Autodesk Fusion 360 part; units mm, degrees
(part 4 of 6)
  spline S137 degree 5 poles (-9.0895, 3.5778) (-9.0878, 3.5785) (-9.078, 3.5823) (-9.0601, 3.5894) (-9.0342, 3.5998) (-9.0002, 3.6135) (-8.9599, 3.6301) (-8.9196, 3.6469) (-8.8794, 3.6639) (-8.8392, 3.6811) (-8.799, 3.6985) (-8.759, 3.7161) (-8.7189, 3.734) (-8.6789, 3.752) (-8.639, 3.7703) (-8.5991, 3.7887) (-8.5592, 3.8074) (-8.5194, 3.8262) (-8.4796, 3.8453) (-8.4399, 3.8645) (-8.4002, 3.8839) (-8.3606, 3.9035) (-8.321, 3.9233) (-8.2815, 3.9432) (-8.242, 3.9634) (-8.2025, 3.9837) (-8.1631, 4.0042) (-8.1238, 4.0248) (-8.0844, 4.0457) (-8.0452, 4.0667) (-8.006, 4.0879) (-7.9668, 4.1093) (-7.9277, 4.1308) (-7.8886, 4.1525) (-7.8495, 4.1743) (-7.8105, 4.1963) (-7.7716, 4.2185) (-7.7327, 4.2409) (-7.6938, 4.2634) (-7.655, 4.286) (-7.6163, 4.3089) (-7.5776, 4.3318) (-7.5389, 4.355) (-7.5003, 4.3783) (-7.4617, 4.4017) (-7.4232, 4.4253) (-7.3847, 4.449) (-7.3539, 4.4682) (-7.3309, 4.4826) (-7.3155, 4.4922) (-7.3078, 4.497) knots 0.354152 0.354152 0.354152 0.354152 0.354152 0.354152 0.357143 0.371429 0.385714 0.4 0.414286 0.428571 0.442857 0.457143 0.471429 0.485714 0.5 0.514286 0.528571 0.542857 0.557143 0.571429 0.585714 0.6 0.614286 0.628571 0.642857 0.657143 0.671429 0.685714 0.7 0.714286 0.728571 0.742857 0.757143 0.771429 0.785714 0.8 0.814286 0.828571 0.842857 0.857143 0.871429 0.885714 0.9 0.914286 0.928571 0.942857 0.957143 0.971429 0.985714 1 1 1 1 1 1
  arc A69 (-7.3078, 4.497) -> (-7.4124, 5.2009) centre (-40, 0) ccw
  spline S138 degree 5 poles (-7.4124, 5.2009) (-7.4212, 5.2033) (-7.4386, 5.208) (-7.4649, 5.2151) (-7.4999, 5.2245) (-7.5436, 5.236) (-7.5873, 5.2474) (-7.631, 5.2586) (-7.6748, 5.2696) (-7.7185, 5.2805) (-7.7622, 5.2913) (-7.8059, 5.3018) (-7.8497, 5.3122) (-7.8934, 5.3225) (-7.9371, 5.3325) (-7.9808, 5.3424) (-8.0245, 5.3522) (-8.0682, 5.3617) (-8.1119, 5.3711) (-8.1556, 5.3803) (-8.1993, 5.3894) (-8.243, 5.3983) (-8.2867, 5.4069) (-8.3303, 5.4155) (-8.374, 5.4238) (-8.4177, 5.432) (-8.4613, 5.4399) (-8.505, 5.4477) (-8.5486, 5.4553) (-8.5922, 5.4627) (-8.6358, 5.47) (-8.6794, 5.477) (-8.723, 5.4838) (-8.7666, 5.4905) (-8.8102, 5.4969) (-8.8538, 5.5032) (-8.8973, 5.5093) (-8.9408, 5.5151) (-8.9844, 5.5207) (-9.0279, 5.5262) (-9.0713, 5.5314) (-9.1148, 5.5364) (-9.1583, 5.5412) (-9.2017, 5.5458) (-9.2451, 5.5501) (-9.2885, 5.5543) (-9.325, 5.5575) (-9.3529, 5.5599) (-9.372, 5.5615) (-9.3825, 5.5623) (-9.3843, 5.5625) knots -1 -1 -1 -1 -1 -1 -0.985714 -0.971429 -0.957143 -0.942857 -0.928571 -0.914286 -0.9 -0.885714 -0.871429 -0.857143 -0.842857 -0.828571 -0.814286 -0.8 -0.785714 -0.771429 -0.757143 -0.742857 -0.728571 -0.714286 -0.7 -0.685714 -0.671429 -0.657143 -0.642857 -0.628571 -0.614286 -0.6 -0.585714 -0.571429 -0.557143 -0.542857 -0.528571 -0.514286 -0.5 -0.485714 -0.471429 -0.457143 -0.442857 -0.428571 -0.414286 -0.4 -0.385714 -0.371429 -0.357143 -0.354152 -0.354152 -0.354152 -0.354152 -0.354152 -0.354152
  spline S139 degree 3 poles (-9.8347, 5.9639) (-9.8221, 5.9) (-9.7971, 5.8392) (-9.7252, 5.7306) (-9.679, 5.6839) (-9.5895, 5.6231) (-9.5509, 5.6036) (-9.4696, 5.5749) (-9.4273, 5.5659) (-9.3843, 5.5625) knots 0 0 0 0 0.019532 0.019532 0.039064 0.039064 0.051994 0.051994 0.064924 0.064924 0.064924 0.064924
  arc A70 (-9.8347, 5.9639) -> (-9.8512, 6.047) centre (-40, 0) ccw
  spline S140 degree 3 poles (-9.589, 6.5903) (-9.6469, 6.5606) (-9.6985, 6.5199) (-9.7832, 6.421) (-9.8155, 6.3637) (-9.8494, 6.261) (-9.8575, 6.2185) (-9.8627, 6.1324) (-9.8597, 6.0892) (-9.8512, 6.047) knots 0 0 0 0 0.019532 0.019532 0.039064 0.039064 0.051994 0.051994 0.064924 0.064924 0.064924 0.064924
  spline S141 degree 5 poles (-9.589, 6.5903) (-9.5874, 6.5912) (-9.578, 6.5959) (-9.5609, 6.6047) (-9.5361, 6.6176) (-9.5036, 6.6346) (-9.4651, 6.6551) (-9.4267, 6.6757) (-9.3883, 6.6966) (-9.35, 6.7176) (-9.3118, 6.7389) (-9.2736, 6.7604) (-9.2355, 6.7821) (-9.1975, 6.804) (-9.1595, 6.8261) (-9.1216, 6.8483) (-9.0838, 6.8708) (-9.046, 6.8934) (-9.0083, 6.9163) (-8.9707, 6.9393) (-8.9331, 6.9625) (-8.8955, 6.9859) (-8.8581, 7.0095) (-8.8207, 7.0332) (-8.7834, 7.0571) (-8.7461, 7.0812) (-8.7089, 7.1055) (-8.6718, 7.1299) (-8.6347, 7.1545) (-8.5977, 7.1792) (-8.5607, 7.2042) (-8.5238, 7.2293) (-8.487, 7.2545) (-8.4502, 7.2799) (-8.4135, 7.3055) (-8.3769, 7.3313) (-8.3403, 7.3571) (-8.3037, 7.3832) (-8.2673, 7.4094) (-8.2309, 7.4358) (-8.1945, 7.4623) (-8.1583, 7.4889) (-8.1221, 7.5157) (-8.0859, 7.5427) (-8.0498, 7.5698) (-8.0138, 7.5971) (-7.9778, 7.6245) (-7.9491, 7.6465) (-7.9276, 7.6631) (-7.9132, 7.6742) (-7.9061, 7.6798) knots 0.354152 0.354152 0.354152 0.354152 0.354152 0.354152 0.357143 0.371429 0.385714 0.4 0.414286 0.428571 0.442857 0.457143 0.471429 0.485714 0.5 0.514286 0.528571 0.542857 0.557143 0.571429 0.585714 0.6 0.614286 0.628571 0.642857 0.657143 0.671429 0.685714 0.7 0.714286 0.728571 0.742857 0.757143 0.771429 0.785714 0.8 0.814286 0.828571 0.842857 0.857143 0.871429 0.885714 0.9 0.914286 0.928571 0.942857 0.957143 0.971429 0.985714 1 1 1 1 1 1
  arc A71 (-7.9061, 7.6798) -> (-8.0791, 8.37) centre (-40, 0) ccw
  spline S142 degree 5 poles (-8.0791, 8.37) (-8.088, 8.3715) (-8.1059, 8.3745) (-8.1327, 8.379) (-8.1684, 8.3849) (-8.2131, 8.3921) (-8.2577, 8.3991) (-8.3023, 8.406) (-8.3469, 8.4127) (-8.3915, 8.4192) (-8.4361, 8.4256) (-8.4806, 8.4319) (-8.5252, 8.4379) (-8.5697, 8.4438) (-8.6142, 8.4496) (-8.6586, 8.4551) (-8.7031, 8.4605) (-8.7475, 8.4658) (-8.7919, 8.4708) (-8.8363, 8.4757) (-8.8807, 8.4804) (-8.925, 8.485) (-8.9694, 8.4894) (-9.0137, 8.4936) (-9.0579, 8.4976) (-9.1022, 8.5014) (-9.1464, 8.5051) (-9.1906, 8.5085) (-9.2348, 8.5118) (-9.2789, 8.5149) (-9.323, 8.5178) (-9.3671, 8.5206) (-9.4112, 8.5231) (-9.4552, 8.5255) (-9.4992, 8.5276) (-9.5431, 8.5296) (-9.5871, 8.5313) (-9.631, 8.5329) (-9.6748, 8.5342) (-9.7187, 8.5354) (-9.7624, 8.5363) (-9.8062, 8.537) (-9.8499, 8.5375) (-9.8936, 8.5378) (-9.9372, 8.5379) (-9.9808, 8.5378) (-10.0175, 8.5375) (-10.0454, 8.5371) (-10.0646, 8.5368) (-10.0751, 8.5366) (-10.0769, 8.5366) knots -1 -1 -1 -1 -1 -1 -0.985714 -0.971429 -0.957143 -0.942857 -0.928571 -0.914286 -0.9 -0.885714 -0.871429 -0.857143 -0.842857 -0.828571 -0.814286 -0.8 -0.785714 -0.771429 -0.757143 -0.742857 -0.728571 -0.714286 -0.7 -0.685714 -0.671429 -0.657143 -0.642857 -0.628571 -0.614286 -0.6 -0.585714 -0.571429 -0.557143 -0.542857 -0.528571 -0.514286 -0.5 -0.485714 -0.471429 -0.457143 -0.442857 -0.428571 -0.414286 -0.4 -0.385714 -0.371429 -0.357143 -0.354152 -0.354152 -0.354152 -0.354152 -0.354152 -0.354152
  spline S143 degree 3 poles (-10.5645, 8.8919) (-10.5457, 8.8296) (-10.5149, 8.7715) (-10.4327, 8.6705) (-10.3822, 8.6285) (-10.2871, 8.5767) (-10.2468, 8.5611) (-10.163, 8.5406) (-10.12, 8.5358) (-10.0769, 8.5366) knots 0 0 0 0 0.019532 0.019532 0.039064 0.039064 0.051994 0.051994 0.064924 0.064924 0.064924 0.064924
  arc A72 (-10.5645, 8.8919) -> (-10.5891, 8.973) centre (-40, 0) ccw
  spline S144 degree 3 poles (-10.3814, 9.5394) (-10.4361, 9.5042) (-10.4835, 9.4586) (-10.5581, 9.3518) (-10.5846, 9.2917) (-10.6082, 9.1861) (-10.6122, 9.143) (-10.6089, 9.0569) (-10.6017, 9.0142) (-10.5891, 8.973) knots 0 0 0 0 0.019532 0.019532 0.039064 0.039064 0.051994 0.051994 0.064924 0.064924 0.064924 0.064924
  spline S145 degree 5 poles (-10.3814, 9.5394) (-10.3799, 9.5404) (-10.371, 9.5461) (-10.3549, 9.5565) (-10.3315, 9.5717) (-10.3008, 9.5918) (-10.2645, 9.6159) (-10.2283, 9.6403) (-10.1921, 9.6648) (-10.1561, 9.6895) (-10.1201, 9.7144) (-10.0842, 9.7396) (-10.0484, 9.7649) (-10.0127, 9.7904) (-9.9771, 9.8161) (-9.9416, 9.842) (-9.9061, 9.868) (-9.8707, 9.8943) (-9.8354, 9.9207) (-9.8002, 9.9473) (-9.7651, 9.9741) (-9.7301, 10.001) (-9.6951, 10.0281) (-9.6602, 10.0554) (-9.6254, 10.0829) (-9.5907, 10.1105) (-9.556, 10.1383) (-9.5215, 10.1663) (-9.487, 10.1944) (-9.4526, 10.2226) (-9.4182, 10.2511) (-9.384, 10.2797) (-9.3498, 10.3084) (-9.3157, 10.3373) (-9.2817, 10.3664) (-9.2477, 10.3956) (-9.2138, 10.4249) (-9.1801, 10.4544) (-9.1463, 10.4841) (-9.1127, 10.5139) (-9.0791, 10.5438) (-9.0456, 10.5739) (-9.0122, 10.6041) (-8.9789, 10.6345) (-8.9456, 10.665) (-8.9124, 10.6957) (-8.8793, 10.7265) (-8.8529, 10.7512) (-8.8331, 10.7699) (-8.8199, 10.7823) (-8.8133, 10.7885) knots 0.354152 0.354152 0.354152 0.354152 0.354152 0.354152 0.357143 0.371429 0.385714 0.4 0.414286 0.428571 0.442857 0.457143 0.471429 0.485714 0.5 0.514286 0.528571 0.542857 0.557143 0.571429 0.585714 0.6 0.614286 0.628571 0.642857 0.657143 0.671429 0.685714 0.7 0.714286 0.728571 0.742857 0.757143 0.771429 0.785714 0.8 0.814286 0.828571 0.842857 0.857143 0.871429 0.885714 0.9 0.914286 0.928571 0.942857 0.957143 0.971429 0.985714 1 1 1 1 1 1
  arc A73 (-8.8133, 10.7885) -> (-9.0532, 11.4585) centre (-40, 0) ccw
  spline S146 degree 5 poles (-9.0532, 11.4585) (-9.0623, 11.4591) (-9.0803, 11.4603) (-9.1074, 11.4622) (-9.1436, 11.4645) (-9.1887, 11.4673) (-9.2338, 11.4699) (-9.2789, 11.4724) (-9.3239, 11.4747) (-9.3689, 11.4769) (-9.4139, 11.4789) (-9.4589, 11.4807) (-9.5038, 11.4824) (-9.5487, 11.4839) (-9.5935, 11.4852) (-9.6383, 11.4864) (-9.6831, 11.4874) (-9.7278, 11.4883) (-9.7725, 11.489) (-9.8171, 11.4895) (-9.8618, 11.4898) (-9.9063, 11.49) (-9.9509, 11.49) (-9.9954, 11.4898) (-10.0398, 11.4895) (-10.0842, 11.489) (-10.1286, 11.4883) (-10.1729, 11.4874) (-10.2172, 11.4864) (-10.2614, 11.4851) (-10.3056, 11.4837) (-10.3498, 11.4821) (-10.3939, 11.4803) (-10.4379, 11.4783) (-10.4819, 11.4762) (-10.5258, 11.4738) (-10.5697, 11.4712) (-10.6136, 11.4685) (-10.6574, 11.4655) (-10.7011, 11.4624) (-10.7447, 11.459) (-10.7884, 11.4554) (-10.8319, 11.4517) (-10.8754, 11.4477) (-10.9188, 11.4435) (-10.9622, 11.4391) (-10.9987, 11.4351) (-11.0264, 11.432) (-11.0455, 11.4299) (-11.056, 11.4286) (-11.0578, 11.4284) knots -1 -1 -1 -1 -1 -1 -0.985714 -0.971429 -0.957143 -0.942857 -0.928571 -0.914286 -0.9 -0.885714 -0.871429 -0.857143 -0.842857 -0.828571 -0.814286 -0.8 -0.785714 -0.771429 -0.757143 -0.742857 -0.728571 -0.714286 -0.7 -0.685714 -0.671429 -0.657143 -0.642857 -0.628571 -0.614286 -0.6 -0.585714 -0.571429 -0.557143 -0.542857 -0.528571 -0.514286 -0.5 -0.485714 -0.471429 -0.457143 -0.442857 -0.428571 -0.414286 -0.4 -0.385714 -0.371429 -0.357143 -0.354152 -0.354152 -0.354152 -0.354152 -0.354152 -0.354152
  spline S147 degree 3 poles (-11.5778, 11.7343) (-11.553, 11.6741) (-11.5166, 11.6193) (-11.4249, 11.5268) (-11.3705, 11.49) (-11.2709, 11.4478) (-11.2292, 11.4362) (-11.1438, 11.424) (-11.1006, 11.4234) (-11.0578, 11.4284) knots 0 0 0 0 0.019532 0.019532 0.039064 0.039064 0.051994 0.051994 0.064924 0.064924 0.064924 0.064924
  arc A74 (-11.5778, 11.7343) -> (-11.6103, 11.8125) centre (-40, 0) ccw
  spline S148 degree 3 poles (-11.459, 12.3966) (-11.5101, 12.3562) (-11.5527, 12.3062) (-11.6165, 12.1926) (-11.637, 12.1302) (-11.6501, 12.0228) (-11.6498, 11.9795) (-11.6382, 11.8941) (-11.6268, 11.8523) (-11.6103, 11.8125) knots 0 0 0 0 0.019532 0.019532 0.039064 0.039064 0.051994 0.051994 0.064924 0.064924 0.064924 0.064924
  spline S149 degree 5 poles (-11.459, 12.3966) (-11.4576, 12.3977) (-11.4494, 12.4042) (-11.4343, 12.4162) (-11.4125, 12.4337) (-11.384, 12.4567) (-11.3502, 12.4842) (-11.3165, 12.512) (-11.283, 12.5399) (-11.2495, 12.5681) (-11.2162, 12.5964) (-11.1829, 12.6249) (-11.1498, 12.6536) (-11.1168, 12.6825) (-11.0838, 12.7116) (-11.051, 12.7408) (-11.0183, 12.7702) (-10.9856, 12.7998) (-10.9531, 12.8296) (-10.9207, 12.8595) (-10.8883, 12.8896) (-10.8561, 12.9198) (-10.824, 12.9503) (-10.7919, 12.9808) (-10.76, 13.0116) (-10.7281, 13.0425) (-10.6964, 13.0735) (-10.6647, 13.1047) (-10.6331, 13.1361) (-10.6016, 13.1676) (-10.5703, 13.1993) (-10.539, 13.2311) (-10.5078, 13.263) (-10.4767, 13.2951) (-10.4457, 13.3274) (-10.4147, 13.3598) (-10.3839, 13.3923) (-10.3532, 13.425) (-10.3225, 13.4578) (-10.292, 13.4907) (-10.2615, 13.5238) (-10.2311, 13.557) (-10.2008, 13.5904) (-10.1706, 13.6239) (-10.1405, 13.6575) (-10.1105, 13.6913) (-10.0806, 13.7252) (-10.0567, 13.7524) (-10.0388, 13.7729) (-10.0269, 13.7866) (-10.021, 13.7934) knots 0.354152 0.354152 0.354152 0.354152 0.354152 0.354152 0.357143 0.371429 0.385714 0.4 0.414286 0.428571 0.442857 0.457143 0.471429 0.485714 0.5 0.514286 0.528571 0.542857 0.557143 0.571429 0.585714 0.6 0.614286 0.628571 0.642857 0.657143 0.671429 0.685714 0.7 0.714286 0.728571 0.742857 0.757143 0.771429 0.785714 0.8 0.814286 0.828571 0.842857 0.857143 0.871429 0.885714 0.9 0.914286 0.928571 0.942857 0.957143 0.971429 0.985714 1 1 1 1 1 1
  arc A75 (-10.021, 13.7934) -> (-10.3254, 14.4366) centre (-40, 0) ccw
  spline S150 degree 5 poles (-10.3254, 14.4366) (-10.3344, 14.4363) (-10.3525, 14.4358) (-10.3797, 14.435) (-10.4159, 14.4338) (-10.4611, 14.4321) (-10.5062, 14.4303) (-10.5513, 14.4284) (-10.5964, 14.4262) (-10.6414, 14.424) (-10.6863, 14.4215) (-10.7312, 14.419) (-10.7761, 14.4162) (-10.8209, 14.4133) (-10.8657, 14.4103) (-10.9104, 14.4071) (-10.955, 14.4037) (-10.9996, 14.4002) (-11.0442, 14.3965) (-11.0887, 14.3926) (-11.1331, 14.3886) (-11.1775, 14.3844) (-11.2218, 14.38) (-11.2661, 14.3755) (-11.3103, 14.3708) (-11.3544, 14.3659) (-11.3985, 14.3609) (-11.4425, 14.3557) (-11.4865, 14.3503) (-11.5304, 14.3447) (-11.5742, 14.339) (-11.618, 14.333) (-11.6617, 14.3269) (-11.7053, 14.3206) (-11.7489, 14.3142) (-11.7924, 14.3075) (-11.8358, 14.3007) (-11.8792, 14.2936) (-11.9225, 14.2864) (-11.9657, 14.279) (-12.0088, 14.2713) (-12.0518, 14.2635) (-12.0948, 14.2555) (-12.1377, 14.2473) (-12.1805, 14.2388) (-12.2233, 14.2302) (-12.2591, 14.2227) (-12.2865, 14.2169) (-12.3053, 14.2129) (-12.3155, 14.2106) (-12.3173, 14.2102) knots -1 -1 -1 -1 -1 -1 -0.985714 -0.971429 -0.957143 -0.942857 -0.928571 -0.914286 -0.9 -0.885714 -0.871429 -0.857143 -0.842857 -0.828571 -0.814286 -0.8 -0.785714 -0.771429 -0.757143 -0.742857 -0.728571 -0.714286 -0.7 -0.685714 -0.671429 -0.657143 -0.642857 -0.628571 -0.614286 -0.6 -0.585714 -0.571429 -0.557143 -0.542857 -0.528571 -0.514286 -0.5 -0.485714 -0.471429 -0.457143 -0.442857 -0.428571 -0.414286 -0.4 -0.385714 -0.371429 -0.357143 -0.354152 -0.354152 -0.354152 -0.354152 -0.354152 -0.354152
  spline S151 degree 3 poles (-12.8648, 14.4636) (-12.8342, 14.4062) (-12.7927, 14.3552) (-12.6924, 14.2722) (-12.6346, 14.2409) (-12.5313, 14.2086) (-12.4887, 14.2012) (-12.4025, 14.1974) (-12.3594, 14.2011) (-12.3173, 14.2102) knots 0 0 0 0 0.019532 0.019532 0.039064 0.039064 0.051994 0.051994 0.064924 0.064924 0.064924 0.064924
  arc A76 (-12.8648, 14.4636) -> (-12.9048, 14.5383) centre (-40, 0) ccw
  spline S152 degree 3 poles (-12.8115, 15.1344) (-12.8584, 15.0892) (-12.8959, 15.0352) (-12.9482, 14.916) (-12.9625, 14.8518) (-12.9651, 14.7436) (-12.9606, 14.7006) (-12.9406, 14.6168) (-12.9252, 14.5763) (-12.9048, 14.5383) knots 0 0 0 0 0.019532 0.019532 0.039064 0.039064 0.051994 0.051994 0.064924 0.064924 0.064924 0.064924
  spline S153 degree 5 poles (-12.8115, 15.1344) (-12.8102, 15.1357) (-12.8027, 15.143) (-12.7889, 15.1563) (-12.7689, 15.1758) (-12.7427, 15.2016) (-12.7118, 15.2323) (-12.681, 15.2632) (-12.6504, 15.2943) (-12.6198, 15.3256) (-12.5894, 15.3571) (-12.5591, 15.3887) (-12.529, 15.4205) (-12.4989, 15.4525) (-12.469, 15.4846) (-12.4392, 15.517) (-12.4095, 15.5494) (-12.3799, 15.5821) (-12.3505, 15.6149) (-12.3211, 15.6478) (-12.2919, 15.681) (-12.2628, 15.7142) (-12.2338, 15.7477) (-12.2049, 15.7812) (-12.1761, 15.8149) (-12.1474, 15.8488) (-12.1189, 15.8828) (-12.0904, 15.917) (-12.0621, 15.9513) (-12.0339, 15.9857) (-12.0057, 16.0203) (-11.9777, 16.055) (-11.9498, 16.0899) (-11.922, 16.1249) (-11.8943, 16.16) (-11.8667, 16.1953) (-11.8392, 16.2307) (-11.8118, 16.2662) (-11.7845, 16.3019) (-11.7573, 16.3377) (-11.7303, 16.3736) (-11.7033, 16.4096) (-11.6764, 16.4458) (-11.6496, 16.4821) (-11.623, 16.5185) (-11.5964, 16.5551) (-11.5699, 16.5917) (-11.5488, 16.6212) (-11.5331, 16.6433) (-11.5226, 16.6581) (-11.5173, 16.6655) knots 0.354152 0.354152 0.354152 0.354152 0.354152 0.354152 0.357143 0.371429 0.385714 0.4 0.414286 0.428571 0.442857 0.457143 0.471429 0.485714 0.5 0.514286 0.528571 0.542857 0.557143 0.571429 0.585714 0.6 0.614286 0.628571 0.642857 0.657143 0.671429 0.685714 0.7 0.714286 0.728571 0.742857 0.757143 0.771429 0.785714 0.8 0.814286 0.828571 0.842857 0.857143 0.871429 0.885714 0.9 0.914286 0.928571 0.942857 0.957143 0.971429 0.985714 1 1 1 1 1 1
  arc A77 (-11.5173, 16.6655) -> (-11.8833, 17.2757) centre (-40, 0) ccw
  spline S154 degree 5 poles (-11.8833, 17.2757) (-11.8923, 17.2746) (-11.9103, 17.2723) (-11.9372, 17.2688) (-11.9731, 17.264) (-12.0179, 17.258) (-12.0627, 17.2517) (-12.1073, 17.2454) (-12.152, 17.2388) (-12.1965, 17.2322) (-12.241, 17.2253) (-12.2855, 17.2184) (-12.3299, 17.2113) (-12.3742, 17.204) (-12.4184, 17.1966) (-12.4626, 17.189) (-12.5067, 17.1812) (-12.5507, 17.1734) (-12.5947, 17.1653) (-12.6386, 17.1571) (-12.6824, 17.1487) (-12.7262, 17.1402) (-12.7699, 17.1315) (-12.8135, 17.1227) (-12.857, 17.1137) (-12.9005, 17.1045) (-12.9438, 17.0952) (-12.9871, 17.0857) (-13.0304, 17.076) (-13.0735, 17.0661) (-13.1166, 17.0561) (-13.1595, 17.0459) (-13.2024, 17.0356) (-13.2452, 17.025) (-13.288, 17.0143) (-13.3306, 17.0034) (-13.3732, 16.9924) (-13.4156, 16.9811) (-13.458, 16.9697) (-13.5002, 16.9581) (-13.5424, 16.9462) (-13.5845, 16.9342) (-13.6265, 16.922) (-13.6684, 16.9096) (-13.7101, 16.897) (-13.7518, 16.8842) (-13.7868, 16.8733) (-13.8134, 16.8648) (-13.8317, 16.859) (-13.8417, 16.8557) (-13.8435, 16.8552) knots -1 -1 -1 -1 -1 -1 -0.985714 -0.971429 -0.957143 -0.942857 -0.928571 -0.914286 -0.9 -0.885714 -0.871429 -0.857143 -0.842857 -0.828571 -0.814286 -0.8 -0.785714 -0.771429 -0.757143 -0.742857 -0.728571 -0.714286 -0.7 -0.685714 -0.671429 -0.657143 -0.642857 -0.628571 -0.614286 -0.6 -0.585714 -0.571429 -0.557143 -0.542857 -0.528571 -0.514286 -0.5 -0.485714 -0.471429 -0.457143 -0.442857 -0.428571 -0.414286 -0.4 -0.385714 -0.371429 -0.357143 -0.354152 -0.354152 -0.354152 -0.354152 -0.354152 -0.354152
  spline S155 degree 3 poles (-14.4132, 17.0537) (-14.3771, 16.9995) (-14.3307, 16.9529) (-14.2228, 16.8801) (-14.1622, 16.8546) (-14.0563, 16.8326) (-14.0131, 16.8294) (-13.927, 16.8341) (-13.8845, 16.8419) (-13.8435, 16.8552) knots 0 0 0 0 0.019532 0.019532 0.039064 0.039064 0.051994 0.051994 0.064924 0.064924 0.064924 0.064924
  arc A78 (-14.4132, 17.0537) -> (-14.4603, 17.1241) centre (-40, 0) ccw
  spline S156 degree 3 poles (-14.4259, 17.7265) (-14.4681, 17.6769) (-14.5002, 17.6195) (-14.5405, 17.4957) (-14.5484, 17.4304) (-14.5404, 17.3225) (-14.5317, 17.2801) (-14.5035, 17.1987) (-14.4843, 17.1599) (-14.4603, 17.1241) knots 0 0 0 0 0.019532 0.019532 0.039064 0.039064 0.051994 0.051994 0.064924 0.064924 0.064924 0.064924
  spline S157 degree 5 poles (-14.4259, 17.7265) (-14.4247, 17.7278) (-14.4179, 17.7359) (-14.4055, 17.7505) (-14.3875, 17.7719) (-14.364, 17.8) (-14.3362, 17.8337) (-14.3086, 17.8674) (-14.2812, 17.9014) (-14.2539, 17.9355) (-14.2267, 17.9698) (-14.1996, 18.0043) (-14.1727, 18.0389) (-14.146, 18.0737) (-14.1193, 18.1086) (-14.0928, 18.1437) (-14.0665, 18.1789) (-14.0402, 18.2143) (-14.0141, 18.2498) (-13.9882, 18.2855) (-13.9623, 18.3213) (-13.9366, 18.3573) (-13.911, 18.3934) (-13.8856, 18.4296) (-13.8602, 18.466) (-13.835, 18.5025) (-13.8099, 18.5392) (-13.785, 18.576) (-13.7601, 18.6129) (-13.7354, 18.6499) (-13.7108, 18.6871) (-13.6863, 18.7244) (-13.662, 18.7618) (-13.6377, 18.7994) (-13.6136, 18.837) (-13.5896, 18.8748) (-13.5657, 18.9128) (-13.5419, 18.9508) (-13.5183, 18.989) (-13.4947, 19.0273) (-13.4713, 19.0657) (-13.448, 19.1042) (-13.4248, 19.1428) (-13.4017, 19.1815) (-13.3787, 19.2204) (-13.3559, 19.2594) (-13.3331, 19.2985) (-13.315, 19.3298) (-13.3015, 19.3534) (-13.2925, 19.3691) (-13.288, 19.377) knots 0.354152 0.354152 0.354152 0.354152 0.354152 0.354152 0.357143 0.371429 0.385714 0.4 0.414286 0.428571 0.442857 0.457143 0.471429 0.485714 0.5 0.514286 0.528571 0.542857 0.557143 0.571429 0.585714 0.6 0.614286 0.628571 0.642857 0.657143 0.671429 0.685714 0.7 0.714286 0.728571 0.742857 0.757143 0.771429 0.785714 0.8 0.814286 0.828571 0.842857 0.857143 0.871429 0.885714 0.9 0.914286 0.928571 0.942857 0.957143 0.971429 0.985714 1 1 1 1 1 1
  arc A79 (-13.288, 19.377) -> (-13.712, 19.9484) centre (-40, 0) ccw
  spline S158 degree 5 poles (-13.712, 19.9484) (-13.7208, 19.9464) (-13.7385, 19.9424) (-13.765, 19.9363) (-13.8002, 19.928) (-13.8442, 19.9176) (-13.8882, 19.907) (-13.932, 19.8963) (-13.9758, 19.8854) (-14.0195, 19.8744) (-14.0631, 19.8633) (-14.1066, 19.852) (-14.1501, 19.8405) (-14.1935, 19.8289) (-14.2368, 19.8172) (-14.28, 19.8053) (-14.3231, 19.7933) (-14.3662, 19.7812) (-14.4092, 19.7688) (-14.452, 19.7564) (-14.4948, 19.7438) (-14.5375, 19.731) (-14.5802, 19.7181) (-14.6227, 19.705) (-14.6651, 19.6917) (-14.7075, 19.6784) (-14.7497, 19.6648) (-14.7919, 19.6511) (-14.834, 19.6372) (-14.8759, 19.6232) (-14.9178, 19.609) (-14.9596, 19.5947) (-15.0013, 19.5802) (-15.0428, 19.5655) (-15.0843, 19.5506) (-15.1257, 19.5356) (-15.1669, 19.5204) (-15.2081, 19.5051) (-15.2491, 19.4895) (-15.29, 19.4738) (-15.3308, 19.4579) (-15.3715, 19.4419) (-15.4121, 19.4256) (-15.4526, 19.4092) (-15.4929, 19.3925) (-15.5331, 19.3757) (-15.5669, 19.3614) (-15.5926, 19.3504) (-15.6102, 19.3427) (-15.6198, 19.3385) (-15.6215, 19.3378) knots -1 -1 -1 -1 -1 -1 -0.985714 -0.971429 -0.957143 -0.942857 -0.928571 -0.914286 -0.9 -0.885714 -0.871429 -0.857143 -0.842857 -0.828571 -0.814286 -0.8 -0.785714 -0.771429 -0.757143 -0.742857 -0.728571 -0.714286 -0.7 -0.685714 -0.671429 -0.657143 -0.642857 -0.628571 -0.614286 -0.6 -0.585714 -0.571429 -0.557143 -0.542857 -0.528571 -0.514286 -0.5 -0.485714 -0.471429 -0.457143 -0.442857 -0.428571 -0.414286 -0.4 -0.385714 -0.371429 -0.357143 -0.354152 -0.354152 -0.354152 -0.354152 -0.354152 -0.354152
  spline S159 degree 3 poles (-16.2079, 19.4795) (-16.1667, 19.4291) (-16.116, 19.3873) (-16.0014, 19.3254) (-15.9387, 19.3059) (-15.8311, 19.2945) (-15.7878, 19.2955) (-15.7026, 19.3086) (-15.661, 19.3206) (-15.6215, 19.3378) knots 0 0 0 0 0.019532 0.019532 0.039064 0.039064 0.051994 0.051994 0.064924 0.064924 0.064924 0.064924
  arc A80 (-16.2079, 19.4795) -> (-16.2617, 19.545) centre (-40, 0) ccw
  spline S160 degree 3 poles (-16.2865, 20.1478) (-16.3236, 20.0943) (-16.35, 20.0341) (-16.378, 19.9069) (-16.3795, 19.8412) (-16.3609, 19.7346) (-16.3481, 19.6933) (-16.3121, 19.6149) (-16.2891, 19.5783) (-16.2617, 19.545) knots 0 0 0 0 0.019532 0.019532 0.039064 0.039064 0.051994 0.051994 0.064924 0.064924 0.064924 0.064924
  spline S161 degree 5 poles (-16.2865, 20.1478) (-16.2855, 20.1493) (-16.2795, 20.1579) (-16.2686, 20.1737) (-16.2528, 20.1968) (-16.2322, 20.2271) (-16.2078, 20.2633) (-16.1837, 20.2996) (-16.1597, 20.3361) (-16.1358, 20.3727) (-16.1121, 20.4095) (-16.0886, 20.4465) (-16.0652, 20.4835) (-16.042, 20.5208) (-16.0189, 20.5581) (-15.996, 20.5957) (-15.9732, 20.6333) (-15.9506, 20.6711) (-15.9281, 20.709) (-15.9057, 20.7471) (-15.8835, 20.7852) (-15.8615, 20.8235) (-15.8395, 20.862) (-15.8177, 20.9005) (-15.7961, 20.9392) (-15.7746, 20.978) (-15.7532, 21.017) (-15.732, 21.056) (-15.7109, 21.0952) (-15.6899, 21.1345) (-15.669, 21.1739) (-15.6483, 21.2134) (-15.6278, 21.2531) (-15.6073, 21.2928) (-15.587, 21.3327) (-15.5668, 21.3726) (-15.5467, 21.4127) (-15.5268, 21.4529) (-15.507, 21.4932) (-15.4873, 21.5336) (-15.4678, 21.5741) (-15.4484, 21.6147) (-15.4291, 21.6555) (-15.4099, 21.6963) (-15.3908, 21.7372) (-15.3719, 21.7782) (-15.3531, 21.8193) (-15.3381, 21.8523) (-15.327, 21.8771) (-15.3196, 21.8936) (-15.3159, 21.9019) knots 0.354152 0.354152 0.354152 0.354152 0.354152 0.354152 0.357143 0.371429 0.385714 0.4 0.414286 0.428571 0.442857 0.457143 0.471429 0.485714 0.5 0.514286 0.528571 0.542857 0.557143 0.571429 0.585714 0.6 0.614286 0.628571 0.642857 0.657143 0.671429 0.685714 0.7 0.714286 0.728571 0.742857 0.757143 0.771429 0.785714 0.8 0.814286 0.828571 0.842857 0.857143 0.871429 0.885714 0.9 0.914286 0.928571 0.942857 0.957143 0.971429 0.985714 1 1 1 1 1 1
  arc A81 (-15.3159, 21.9019) -> (-15.7939, 22.4291) centre (-40, 0) ccw
  spline S162 degree 5 poles (-15.7939, 22.4291) (-15.8025, 22.4262) (-15.8196, 22.4204) (-15.8454, 22.4117) (-15.8797, 22.4001) (-15.9224, 22.3854) (-15.9651, 22.3705) (-16.0077, 22.3556) (-16.0502, 22.3405) (-16.0926, 22.3252) (-16.1349, 22.3099) (-16.1771, 22.2944) (-16.2193, 22.2787) (-16.2613, 22.2629) (-16.3033, 22.247) (-16.3451, 22.231) (-16.3869, 22.2148) (-16.4285, 22.1985) (-16.4701, 22.182) (-16.5115, 22.1654) (-16.5529, 22.1486) (-16.5941, 22.1317) (-16.6353, 22.1147) (-16.6763, 22.0975) (-16.7173, 22.0802) (-16.7581, 22.0627) (-16.7988, 22.0451) (-16.8394, 22.0273) (-16.8799, 22.0094) (-16.9203, 21.9913) (-16.9606, 21.9731) (-17.0008, 21.9547) (-17.0408, 21.9362) (-17.0808, 21.9175) (-17.1206, 21.8987) (-17.1603, 21.8797) (-17.1998, 21.8605) (-17.2393, 21.8412) (-17.2786, 21.8217) (-17.3178, 21.8021) (-17.3568, 21.7822) (-17.3958, 21.7623) (-17.4346, 21.7421) (-17.4732, 21.7218) (-17.5117, 21.7013) (-17.5501, 21.6806) (-17.5823, 21.663) (-17.6068, 21.6495) (-17.6236, 21.6402) (-17.6327, 21.6351) (-17.6343, 21.6342) knots -1 -1 -1 -1 -1 -1 -0.985714 -0.971429 -0.957143 -0.942857 -0.928571 -0.914286 -0.9 -0.885714 -0.871429 -0.857143 -0.842857 -0.828571 -0.814286 -0.8 -0.785714 -0.771429 -0.757143 -0.742857 -0.728571 -0.714286 -0.7 -0.685714 -0.671429 -0.657143 -0.642857 -0.628571 -0.614286 -0.6 -0.585714 -0.571429 -0.557143 -0.542857 -0.528571 -0.514286 -0.5 -0.485714 -0.471429 -0.457143 -0.442857 -0.428571 -0.414286 -0.4 -0.385714 -0.371429 -0.357143 -0.354152 -0.354152 -0.354152 -0.354152 -0.354152 -0.354152
  spline S163 degree 3 poles (-18.2318, 21.7177) (-18.1859, 21.6717) (-18.1313, 21.635) (-18.0112, 21.5846) (-17.9468, 21.5714) (-17.8386, 21.5706) (-17.7957, 21.5758) (-17.7122, 21.5972) (-17.672, 21.6132) (-17.6343, 21.6342) knots 0 0 0 0 0.019532 0.019532 0.039064 0.039064 0.051994 0.051994 0.064924 0.064924 0.064924 0.064924
  arc A82 (-18.2318, 21.7177) -> (-18.2918, 21.7776) centre (-40, 0) ccw
  spline S164 degree 3 poles (-18.3756, 22.3751) (-18.4072, 22.3182) (-18.4275, 22.2557) (-18.443, 22.1264) (-18.438, 22.0609) (-18.4091, 21.9566) (-18.3922, 21.9167) (-18.3487, 21.8423) (-18.3223, 21.8081) (-18.2918, 21.7776) knots 0 0 0 0 0.019532 0.019532 0.039064 0.039064 0.051994 0.051994 0.064924 0.064924 0.064924 0.064924
  spline S165 degree 5 poles (-18.3756, 22.3751) (-18.3747, 22.3767) (-18.3695, 22.3859) (-18.3602, 22.4027) (-18.3468, 22.4272) (-18.3292, 22.4593) (-18.3085, 22.4977) (-18.2881, 22.5363) (-18.2678, 22.5749) (-18.2476, 22.6137) (-18.2276, 22.6527) (-18.2078, 22.6917) (-18.1882, 22.7309) (-18.1687, 22.7703) (-18.1494, 22.8097) (-18.1303, 22.8493) (-18.1113, 22.889) (-18.0925, 22.9288) (-18.0738, 22.9687) (-18.0553, 23.0088) (-18.037, 23.049) (-18.0188, 23.0893) (-18.0007, 23.1297) (-17.9828, 23.1702) (-17.965, 23.2108) (-17.9474, 23.2515) (-17.93, 23.2924) (-17.9127, 23.3333) (-17.8955, 23.3744) (-17.8785, 23.4155) (-17.8616, 23.4568) (-17.8449, 23.4982) (-17.8283, 23.5396) (-17.8118, 23.5812) (-17.7955, 23.6228) (-17.7793, 23.6646) (-17.7633, 23.7064) (-17.7474, 23.7484) (-17.7317, 23.7904) (-17.716, 23.8326) (-17.7005, 23.8748) (-17.6852, 23.9171) (-17.67, 23.9595) (-17.6549, 24.0021) (-17.6399, 24.0446) (-17.6251, 24.0873) (-17.6104, 24.1301) (-17.5988, 24.1644) (-17.5901, 24.1901) (-17.5844, 24.2073) (-17.5815, 24.2159) knots 0.354152 0.354152 0.354152 0.354152 0.354152 0.354152 0.357143 0.371429 0.385714 0.4 0.414286 0.428571 0.442857 0.457143 0.471429 0.485714 0.5 0.514286 0.528571 0.542857 0.557143 0.571429 0.585714 0.6 0.614286 0.628571 0.642857 0.657143 0.671429 0.685714 0.7 0.714286 0.728571 0.742857 0.757143 0.771429 0.785714 0.8 0.814286 0.828571 0.842857 0.857143 0.871429 0.885714 0.9 0.914286 0.928571 0.942857 0.957143 0.971429 0.985714 1 1 1 1 1 1
  arc A83 (-17.5815, 24.2159) -> (-18.1088, 24.6937) centre (-40, 0) ccw
  spline S166 degree 5 poles (-18.1088, 24.6937) (-18.1171, 24.69) (-18.1337, 24.6826) (-18.1584, 24.6714) (-18.1914, 24.6564) (-18.2325, 24.6376) (-18.2735, 24.6187) (-18.3145, 24.5996) (-18.3553, 24.5804) (-18.396, 24.5611) (-18.4366, 24.5416) (-18.4771, 24.5221) (-18.5175, 24.5024) (-18.5578, 24.4825) (-18.598, 24.4626) (-18.638, 24.4425) (-18.678, 24.4223) (-18.7178, 24.402) (-18.7576, 24.3815) (-18.7972, 24.3609) (-18.8367, 24.3402) (-18.8761, 24.3193) (-18.9154, 24.2983) (-18.9546, 24.2772) (-18.9936, 24.256) (-19.0325, 24.2346) (-19.0713, 24.213) (-19.11, 24.1914) (-19.1486, 24.1696) (-19.187, 24.1476) (-19.2253, 24.1255) (-19.2635, 24.1033) (-19.3015, 24.081) (-19.3394, 24.0585) (-19.3772, 24.0358) (-19.4148, 24.013) (-19.4523, 23.9901) (-19.4897, 23.967) (-19.5269, 23.9437) (-19.564, 23.9203) (-19.6009, 23.8968) (-19.6377, 23.8731) (-19.6743, 23.8492) (-19.7108, 23.8252) (-19.7471, 23.801) (-19.7833, 23.7767) (-19.8136, 23.756) (-19.8366, 23.7402) (-19.8524, 23.7293) (-19.8611, 23.7233) (-19.8626, 23.7223) knots -1 -1 -1 -1 -1 -1 -0.985714 -0.971429 -0.957143 -0.942857 -0.928571 -0.914286 -0.9 -0.885714 -0.871429 -0.857143 -0.842857 -0.828571 -0.814286 -0.8 -0.785714 -0.771429 -0.757143 -0.742857 -0.728571 -0.714286 -0.7 -0.685714 -0.671429 -0.657143 -0.642857 -0.628571 -0.614286 -0.6 -0.585714 -0.571429 -0.557143 -0.542857 -0.528571 -0.514286 -0.5 -0.485714 -0.471429 -0.457143 -0.442857 -0.428571 -0.414286 -0.4 -0.385714 -0.371429 -0.357143 -0.354152 -0.354152 -0.354152 -0.354152 -0.354152 -0.354152
  spline S167 degree 3 poles (-20.4654, 23.7468) (-20.4151, 23.7055) (-20.3572, 23.6743) (-20.2328, 23.636) (-20.1674, 23.6291) (-20.0596, 23.6389) (-20.0174, 23.6483) (-19.9364, 23.6778) (-19.898, 23.6977) (-19.8626, 23.7223) knots 0 0 0 0 0.019532 0.019532 0.039064 0.039064 0.051994 0.051994 0.064924 0.064924 0.064924 0.064924
  arc A84 (-20.4654, 23.7468) -> (-20.5309, 23.8006) centre (-40, 0) ccw
  spline S168 degree 3 poles (-20.6728, 24.3869) (-20.6988, 24.3272) (-20.7128, 24.263) (-20.7155, 24.1328) (-20.7042, 24.0681) (-20.6652, 23.9672) (-20.6445, 23.9291) (-20.5939, 23.8593) (-20.5642, 23.8278) (-20.5309, 23.8006) knots 0 0 0 0 0.019532 0.019532 0.039064 0.039064 0.051994 0.051994 0.064924 0.064924 0.064924 0.064924
  spline S169 degree 5 poles (-20.6728, 24.3869) (-20.6721, 24.3886) (-20.6679, 24.3982) (-20.6603, 24.4159) (-20.6493, 24.4416) (-20.635, 24.4753) (-20.6182, 24.5155) (-20.6015, 24.5559) (-20.5851, 24.5964) (-20.5689, 24.6369) (-20.5528, 24.6776) (-20.537, 24.7185) (-20.5213, 24.7594) (-20.5057, 24.8004) (-20.4904, 24.8416) (-20.4752, 24.8829) (-20.4602, 24.9242) (-20.4454, 24.9657) (-20.4307, 25.0073) (-20.4162, 25.049) (-20.4019, 25.0907) (-20.3877, 25.1326) (-20.3737, 25.1746) (-20.3599, 25.2167) (-20.3462, 25.2588) (-20.3327, 25.3011) (-20.3193, 25.3435) (-20.3061, 25.3859) (-20.293, 25.4284) (-20.2801, 25.4711) (-20.2674, 25.5138) (-20.2548, 25.5566) (-20.2423, 25.5995) (-20.23, 25.6424) (-20.2179, 25.6855) (-20.2059, 25.7286) (-20.194, 25.7719) (-20.1823, 25.8152) (-20.1708, 25.8586) (-20.1593, 25.902) (-20.1481, 25.9456) (-20.1369, 25.9892) (-20.126, 26.0329) (-20.1151, 26.0767) (-20.1044, 26.1205) (-20.0938, 26.1645) (-20.0834, 26.2085) (-20.0752, 26.2437) (-20.0691, 26.2702) (-20.065, 26.2879) (-20.063, 26.2967) knots 0.354152 0.354152 0.354152 0.354152 0.354152 0.354152 0.357143 0.371429 0.385714 0.4 0.414286 0.428571 0.442857 0.457143 0.471429 0.485714 0.5 0.514286 0.528571 0.542857 0.557143 0.571429 0.585714 0.6 0.614286 0.628571 0.642857 0.657143 0.671429 0.685714 0.7 0.714286 0.728571 0.742857 0.757143 0.771429 0.785714 0.8 0.814286 0.828571 0.842857 0.857143 0.871429 0.885714 0.9 0.914286 0.928571 0.942857 0.957143 0.971429 0.985714 1 1 1 1 1 1
  arc A85 (-20.063, 26.2967) -> (-20.6347, 26.7205) centre (-40, 0) ccw
  spline S170 degree 5 poles (-20.6347, 26.7205) (-20.6425, 26.716) (-20.6583, 26.707) (-20.6818, 26.6934) (-20.7132, 26.6753) (-20.7523, 26.6525) (-20.7912, 26.6297) (-20.8301, 26.6067) (-20.8688, 26.5836) (-20.9074, 26.5604) (-20.9459, 26.537) (-20.9843, 26.5136) (-21.0226, 26.49) (-21.0607, 26.4664) (-21.0988, 26.4426) (-21.1367, 26.4187) (-21.1745, 26.3946) (-21.2121, 26.3705) (-21.2497, 26.3462) (-21.2871, 26.3219) (-21.3244, 26.2974) (-21.3615, 26.2727) (-21.3986, 26.248) (-21.4355, 26.2231) (-21.4723, 26.1982) (-21.5089, 26.173) (-21.5454, 26.1478) (-21.5818, 26.1225) (-21.618, 26.097) (-21.6541, 26.0714) (-21.69, 26.0457) (-21.7259, 26.0198) (-21.7615, 25.9938) (-21.797, 25.9677) (-21.8324, 25.9414) (-21.8676, 25.9151) (-21.9027, 25.8886) (-21.9376, 25.8619) (-21.9724, 25.8351) (-22.007, 25.8082) (-22.0414, 25.7812) (-22.0757, 25.754) (-22.1098, 25.7266) (-22.1438, 25.6992) (-22.1775, 25.6715) (-22.2112, 25.6438) (-22.2393, 25.6203) (-22.2607, 25.6023) (-22.2753, 25.5898) (-22.2833, 25.583) (-22.2847, 25.5818) knots -1 -1 -1 -1 -1 -1 -0.985714 -0.971429 -0.957143 -0.942857 -0.928571 -0.914286 -0.9 -0.885714 -0.871429 -0.857143 -0.842857 -0.828571 -0.814286 -0.8 -0.785714 -0.771429 -0.757143 -0.742857 -0.728571 -0.714286 -0.7 -0.685714 -0.671429 -0.657143 -0.642857 -0.628571 -0.614286 -0.6 -0.585714 -0.571429 -0.557143 -0.542857 -0.528571 -0.514286 -0.5 -0.485714 -0.471429 -0.457143 -0.442857 -0.428571 -0.414286 -0.4 -0.385714 -0.371429 -0.357143 -0.354152 -0.354152 -0.354152 -0.354152 -0.354152 -0.354152
  spline S171 degree 3 poles (-22.887, 25.5472) (-22.8329, 25.511) (-22.7723, 25.4856) (-22.6447, 25.4597) (-22.579, 25.4593) (-22.4727, 25.4796) (-22.4316, 25.4931) (-22.3538, 25.5303) (-22.3175, 25.5539) (-22.2847, 25.5818) knots 0 0 0 0 0.019532 0.019532 0.039064 0.039064 0.051994 0.051994 0.064924 0.064924 0.064924 0.064924
  arc A86 (-22.887, 25.5472) -> (-22.9575, 25.5943) centre (-40, 0) ccw
  spline S172 degree 3 poles (-23.1562, 26.1639) (-23.1762, 26.1019) (-23.1839, 26.0367) (-23.1738, 25.9068) (-23.1562, 25.8435) (-23.1075, 25.7469) (-23.0832, 25.7111) (-23.026, 25.6466) (-22.9934, 25.6181) (-22.9575, 25.5943) knots 0 0 0 0 0.019532 0.019532 0.039064 0.039064 0.051994 0.051994 0.064924 0.064924 0.064924 0.064924
  spline S173 degree 5 poles (-23.1562, 26.1639) (-23.1557, 26.1656) (-23.1524, 26.1756) (-23.1466, 26.1939) (-23.1381, 26.2206) (-23.1272, 26.2556) (-23.1144, 26.2972) (-23.1019, 26.339) (-23.0895, 26.3809) (-23.0773, 26.4229) (-23.0653, 26.465) (-23.0535, 26.5072) (-23.0419, 26.5494) (-23.0305, 26.5918) (-23.0192, 26.6343) (-23.0082, 26.6768) (-22.9973, 26.7194) (-22.9866, 26.7622) (-22.9761, 26.805) (-22.9658, 26.8479) (-22.9556, 26.8909) (-22.9456, 26.9339) (-22.9358, 26.9771) (-22.9261, 27.0203) (-22.9166, 27.0636) (-22.9073, 27.107) (-22.8982, 27.1505) (-22.8892, 27.194) (-22.8804, 27.2376) (-22.8717, 27.2813) (-22.8632, 27.3251) (-22.8548, 27.3689) (-22.8467, 27.4128) (-22.8386, 27.4568) (-22.8308, 27.5008) (-22.823, 27.5449) (-22.8155, 27.5891) (-22.8081, 27.6333) (-22.8008, 27.6777) (-22.7937, 27.722) (-22.7868, 27.7665) (-22.78, 27.811) (-22.7733, 27.8555) (-22.7668, 27.9002) (-22.7605, 27.9449) (-22.7543, 27.9896) (-22.7482, 28.0344) (-22.7435, 28.0703) (-22.74, 28.0973) (-22.7377, 28.1153) (-22.7366, 28.1243) knots 0.354152 0.354152 0.354152 0.354152 0.354152 0.354152 0.357143 0.371429 0.385714 0.4 0.414286 0.428571 0.442857 0.457143 0.471429 0.485714 0.5 0.514286 0.528571 0.542857 0.557143 0.571429 0.585714 0.6 0.614286 0.628571 0.642857 0.657143 0.671429 0.685714 0.7 0.714286 0.728571 0.742857 0.757143 0.771429 0.785714 0.8 0.814286 0.828571 0.842857 0.857143 0.871429 0.885714 0.9 0.914286 0.928571 0.942857 0.957143 0.971429 0.985714 1 1 1 1 1 1
  arc A87 (-22.7366, 28.1243) -> (-23.347, 28.4899) centre (-40, 0) ccw
  spline S174 degree 5 poles (-23.347, 28.4899) (-23.3544, 28.4847) (-23.3691, 28.4742) (-23.3913, 28.4584) (-23.4207, 28.4373) (-23.4573, 28.4108) (-23.4939, 28.3842) (-23.5303, 28.3575) (-23.5666, 28.3308) (-23.6027, 28.3039) (-23.6388, 28.2769) (-23.6747, 28.2498) (-23.7104, 28.2226) (-23.7461, 28.1953) (-23.7816, 28.1679) (-23.817, 28.1404) (-23.8522, 28.1128) (-23.8874, 28.085) (-23.9223, 28.0572) (-23.9572, 28.0293) (-23.9919, 28.0013) (-24.0265, 27.9731) (-24.0609, 27.9449) (-24.0952, 27.9165) (-24.1293, 27.888) (-24.1633, 27.8595) (-24.1972, 27.8308) (-24.2309, 27.802) (-24.2645, 27.7731) (-24.2979, 27.7441) (-24.3311, 27.7149) (-24.3642, 27.6857) (-24.3972, 27.6563) (-24.43, 27.6269) (-24.4626, 27.5973) (-24.4951, 27.5676) (-24.5274, 27.5377) (-24.5595, 27.5078) (-24.5915, 27.4777) (-24.6233, 27.4476) (-24.6549, 27.4173) (-24.6863, 27.3868) (-24.7176, 27.3563) (-24.7487, 27.3256) (-24.7796, 27.2948) (-24.8103, 27.2639) (-24.836, 27.2377) (-24.8555, 27.2177) (-24.8689, 27.2039) (-24.8762, 27.1964) (-24.8775, 27.1951) knots -1 -1 -1 -1 -1 -1 -0.985714 -0.971429 -0.957143 -0.942857 -0.928571 -0.914286 -0.9 -0.885714 -0.871429 -0.857143 -0.842857 -0.828571 -0.814286 -0.8 -0.785714 -0.771429 -0.757143 -0.742857 -0.728571 -0.714286 -0.7 -0.685714 -0.671429 -0.657143 -0.642857 -0.628571 -0.614286 -0.6 -0.585714 -0.571429 -0.557143 -0.542857 -0.528571 -0.514286 -0.5 -0.485714 -0.471429 -0.457143 -0.442857 -0.428571 -0.414286 -0.4 -0.385714 -0.371429 -0.357143 -0.354152 -0.354152 -0.354152 -0.354152 -0.354152 -0.354152
  spline S175 degree 3 poles (-25.4735, 27.1015) (-25.4161, 27.0708) (-25.3533, 27.0515) (-25.2237, 27.0382) (-25.1583, 27.0442) (-25.0545, 27.0749) (-25.0149, 27.0923) (-24.9412, 27.137) (-24.9074, 27.164) (-24.8775, 27.1951) knots 0 0 0 0 0.019532 0.019532 0.039064 0.039064 0.051994 0.051994 0.064924 0.064924 0.064924 0.064924
  arc A88 (-25.4735, 27.1015) -> (-25.5482, 27.1415) centre (-40, 0) ccw
  spline S176 degree 3 poles (-25.8018, 27.6889) (-25.8157, 27.6253) (-25.8169, 27.5595) (-25.7942, 27.4313) (-25.7704, 27.3701) (-25.7124, 27.2787) (-25.6847, 27.2454) (-25.6215, 27.1868) (-25.5863, 27.1617) (-25.5482, 27.1415) knots 0 0 0 0 0.019532 0.019532 0.039064 0.039064 0.051994 0.051994 0.064924 0.064924 0.064924 0.064924
  spline S177 degree 5 poles (-25.8018, 27.6889) (-25.8015, 27.6907) (-25.7992, 27.7009) (-25.7952, 27.7197) (-25.7894, 27.7471) (-25.7819, 27.783) (-25.7733, 27.8257) (-25.7649, 27.8685) (-25.7567, 27.9114) (-25.7487, 27.9544) (-25.7409, 27.9974) (-25.7333, 28.0406) (-25.7259, 28.0838) (-25.7186, 28.1271) (-25.7116, 28.1704) (-25.7048, 28.2138) (-25.6982, 28.2573) (-25.6917, 28.3009) (-25.6854, 28.3446) (-25.6793, 28.3883) (-25.6734, 28.432) (-25.6677, 28.4759) (-25.6622, 28.5198) (-25.6568, 28.5637) (-25.6516, 28.6078) (-25.6466, 28.6519) (-25.6417, 28.696) (-25.6371, 28.7402) (-25.6325, 28.7845) (-25.6282, 28.8288) (-25.624, 28.8732) (-25.62, 28.9176) (-25.6162, 28.9621) (-25.6125, 29.0067) (-25.609, 29.0513) (-25.6056, 29.0959) (-25.6024, 29.1406) (-25.5994, 29.1854) (-25.5965, 29.2302) (-25.5938, 29.275) (-25.5912, 29.32) (-25.5888, 29.3649) (-25.5866, 29.4099) (-25.5845, 29.455) (-25.5826, 29.5001) (-25.5808, 29.5452) (-25.5791, 29.5904) (-25.5779, 29.6266) (-25.5771, 29.6538) (-25.5766, 29.6719) (-25.5764, 29.6809) knots 0.354152 0.354152 0.354152 0.354152 0.354152 0.354152 0.357143 0.371429 0.385714 0.4 0.414286 0.428571 0.442857 0.457143 0.471429 0.485714 0.5 0.514286 0.528571 0.542857 0.557143 0.571429 0.585714 0.6 0.614286 0.628571 0.642857 0.657143 0.671429 0.685714 0.7 0.714286 0.728571 0.742857 0.757143 0.771429 0.785714 0.8 0.814286 0.828571 0.842857 0.857143 0.871429 0.885714 0.9 0.914286 0.928571 0.942857 0.957143 0.971429 0.985714 1 1 1 1 1 1
  arc A89 (-25.5764, 29.6809) -> (-26.2197, 29.985) centre (-40, 0) ccw
  spline S178 degree 5 poles (-26.2197, 29.985) (-26.2265, 29.9791) (-26.2402, 29.9672) (-26.2607, 29.9493) (-26.2879, 29.9254) (-26.3217, 29.8955) (-26.3555, 29.8654) (-26.3891, 29.8353) (-26.4226, 29.8051) (-26.4559, 29.7748) (-26.4892, 29.7444) (-26.5222, 29.7139) (-26.5552, 29.6833) (-26.588, 29.6527) (-26.6206, 29.6219) (-26.6532, 29.5911) (-26.6855, 29.5601) (-26.7178, 29.5291) (-26.7499, 29.498) (-26.7818, 29.4668) (-26.8136, 29.4355) (-26.8452, 29.4041) (-26.8767, 29.3726) (-26.9081, 29.341) (-26.9393, 29.3093) (-26.9703, 29.2776) (-27.0012, 29.2457) (-27.0319, 29.2138) (-27.0625, 29.1817) (-27.0929, 29.1495) (-27.1231, 29.1173) (-27.1532, 29.0849) (-27.1831, 29.0525) (-27.2128, 29.02) (-27.2424, 28.9873) (-27.2718, 28.9546) (-27.301, 28.9217) (-27.3301, 28.8888) (-27.359, 28.8557) (-27.3876, 28.8226) (-27.4161, 28.7893) (-27.4445, 28.756) (-27.4726, 28.7225) (-27.5005, 28.6889) (-27.5283, 28.6552) (-27.5558, 28.6215) (-27.5788, 28.5929) (-27.5963, 28.5711) (-27.6082, 28.556) (-27.6147, 28.5478) (-27.6159, 28.5464) knots -1 -1 -1 -1 -1 -1 -0.985714 -0.971429 -0.957143 -0.942857 -0.928571 -0.914286 -0.9 -0.885714 -0.871429 -0.857143 -0.842857 -0.828571 -0.814286 -0.8 -0.785714 -0.771429 -0.757143 -0.742857 -0.728571 -0.714286 -0.7 -0.685714 -0.671429 -0.657143 -0.642857 -0.628571 -0.614286 -0.6 -0.585714 -0.571429 -0.557143 -0.542857 -0.528571 -0.514286 -0.5 -0.485714 -0.471429 -0.457143 -0.442857 -0.428571 -0.414286 -0.4 -0.385714 -0.371429 -0.357143 -0.354152 -0.354152 -0.354152 -0.354152 -0.354152 -0.354152
  spline S179 degree 3 poles (-28.1999, 28.3949) (-28.1397, 28.3699) (-28.0753, 28.3569) (-27.9451, 28.3563) (-27.8806, 28.3688) (-27.7803, 28.4094) (-27.7426, 28.4307) (-27.6736, 28.4824) (-27.6426, 28.5126) (-27.6159, 28.5464) knots 0 0 0 0 0.019532 0.019532 0.039064 0.039064 0.051994 0.051994 0.064924 0.064924 0.064924 0.064924
  arc A90 (-28.1999, 28.3949) -> (-28.2781, 28.4273) centre (-40, 0) ccw
  spline S180 degree 3 poles (-28.5842, 28.9472) (-28.5917, 28.8825) (-28.5865, 28.817) (-28.5513, 28.6917) (-28.5216, 28.633) (-28.455, 28.5478) (-28.4242, 28.5174) (-28.3555, 28.4652) (-28.318, 28.4437) (-28.2781, 28.4273) knots 0 0 0 0 0.019532 0.019532 0.039064 0.039064 0.051994 0.051994 0.064924 0.064924 0.064924 0.064924
  spline S181 degree 5 poles (-28.5842, 28.9472) (-28.584, 28.949) (-28.5828, 28.9595) (-28.5806, 28.9786) (-28.5775, 29.0063) (-28.5736, 29.0428) (-28.5692, 29.0862) (-28.565, 29.1296) (-28.5611, 29.1731) (-28.5573, 29.2166) (-28.5538, 29.2603) (-28.5504, 29.3039) (-28.5473, 29.3476) (-28.5443, 29.3914) (-28.5416, 29.4353) (-28.5391, 29.4792) (-28.5367, 29.5231) (-28.5346, 29.5671) (-28.5326, 29.6111) (-28.5308, 29.6552) (-28.5293, 29.6994) (-28.5279, 29.7436) (-28.5266, 29.7878) (-28.5256, 29.8321) (-28.5247, 29.8764) (-28.5241, 29.9208) (-28.5236, 29.9652) (-28.5232, 30.0096) (-28.5231, 30.0541) (-28.5231, 30.0987) (-28.5233, 30.1432) (-28.5237, 30.1879) (-28.5242, 30.2325) (-28.5249, 30.2772) (-28.5258, 30.3219) (-28.5268, 30.3667) (-28.528, 30.4115) (-28.5294, 30.4564) (-28.5309, 30.5012) (-28.5326, 30.5461) (-28.5345, 30.5911) (-28.5365, 30.6361) (-28.5387, 30.6811) (-28.541, 30.7261) (-28.5435, 30.7712) (-28.5461, 30.8163) (-28.5489, 30.8614) (-28.5513, 30.8975) (-28.5531, 30.9247) (-28.5544, 30.9427) (-28.555, 30.9518) knots 0.354152 0.354152 0.354152 0.354152 0.354152 0.354152 0.357143 0.371429 0.385714 0.4 0.414286 0.428571 0.442857 0.457143 0.471429 0.485714 0.5 0.514286 0.528571 0.542857 0.557143 0.571429 0.585714 0.6 0.614286 0.628571 0.642857 0.657143 0.671429 0.685714 0.7 0.714286 0.728571 0.742857 0.757143 0.771429 0.785714 0.8 0.814286 0.828571 0.842857 0.857143 0.871429 0.885714 0.9 0.914286 0.928571 0.942857 0.957143 0.971429 0.985714 1 1 1 1 1 1
  arc A91 (-28.555, 30.9518) -> (-29.2251, 31.1914) centre (-40, 0) ccw
  spline S182 degree 5 poles (-29.2251, 31.1914) (-29.2313, 31.1848) (-29.2437, 31.1716) (-29.2624, 31.1518) (-29.2871, 31.1254) (-29.3179, 31.0922) (-29.3485, 31.059) (-29.379, 31.0257) (-29.4094, 30.9924) (-29.4396, 30.959) (-29.4697, 30.9255) (-29.4996, 30.8919) (-29.5294, 30.8582) (-29.559, 30.8245) (-29.5885, 30.7907) (-29.6179, 30.7568) (-29.647, 30.7229) (-29.6761, 30.6888) (-29.705, 30.6547) (-29.7337, 30.6205) (-29.7623, 30.5862) (-29.7907, 30.5519) (-29.8189, 30.5175) (-29.847, 30.483) (-29.875, 30.4484) (-29.9028, 30.4137) (-29.9304, 30.379) (-29.9578, 30.3442) (-29.9851, 30.3093) (-30.0122, 30.2743) (-30.0391, 30.2392) (-30.0659, 30.2041) (-30.0925, 30.1689) (-30.1189, 30.1336) (-30.1451, 30.0982) (-30.1712, 30.0627) (-30.197, 30.0272) (-30.2227, 29.9915) (-30.2482, 29.9558) (-30.2735, 29.92) (-30.2986, 29.8841) (-30.3235, 29.8482) (-30.3482, 29.8121) (-30.3727, 29.7759) (-30.397, 29.7397) (-30.4211, 29.7034) (-30.4412, 29.6727) (-30.4564, 29.6493) (-30.4669, 29.6331) (-30.4726, 29.6243) (-30.4735, 29.6228) knots -1 -1 -1 -1 -1 -1 -0.985714 -0.971429 -0.957143 -0.942857 -0.928571 -0.914286 -0.9 -0.885714 -0.871429 -0.857143 -0.842857 -0.828571 -0.814286 -0.8 -0.785714 -0.771429 -0.757143 -0.742857 -0.728571 -0.714286 -0.7 -0.685714 -0.671429 -0.657143 -0.642857 -0.628571 -0.614286 -0.6 -0.585714 -0.571429 -0.557143 -0.542857 -0.528571 -0.514286 -0.5 -0.485714 -0.471429 -0.457143 -0.442857 -0.428571 -0.414286 -0.4 -0.385714 -0.371429 -0.357143 -0.354152 -0.354152 -0.354152 -0.354152 -0.354152 -0.354152
  spline S183 degree 3 poles (-31.0399, 29.4148) (-30.9776, 29.3958) (-30.9122, 29.3892) (-30.7826, 29.4014) (-30.7195, 29.4201) (-30.6237, 29.4703) (-30.5883, 29.4952) (-30.5247, 29.5534) (-30.4968, 29.5865) (-30.4735, 29.6228) knots 0 0 0 0 0.019532 0.019532 0.039064 0.039064 0.051994 0.051994 0.064924 0.064924 0.064924 0.064924
  arc A92 (-31.0399, 29.4148) -> (-31.1209, 29.4394) centre (-40, 0) ccw
  spline S184 degree 3 poles (-31.4765, 29.9268) (-31.4776, 29.8617) (-31.466, 29.797) (-31.4187, 29.6757) (-31.3834, 29.6202) (-31.3088, 29.5419) (-31.2751, 29.5147) (-31.2017, 29.4695) (-31.1622, 29.4518) (-31.1209, 29.4394) knots 0 0 0 0 0.019532 0.019532 0.039064 0.039064 0.051994 0.051994 0.064924 0.064924 0.064924 0.064924
  spline S185 degree 5 poles (-31.4765, 29.9268) (-31.4765, 29.9286) (-31.4763, 29.9391) (-31.476, 29.9583) (-31.4756, 29.9863) (-31.4753, 30.0229) (-31.4752, 30.0665) (-31.4753, 30.1101) (-31.4756, 30.1538) (-31.4761, 30.1975) (-31.4769, 30.2413) (-31.4778, 30.2851) (-31.479, 30.3289) (-31.4804, 30.3728) (-31.4819, 30.4166) (-31.4837, 30.4606) (-31.4857, 30.5045) (-31.4879, 30.5485) (-31.4902, 30.5926) (-31.4928, 30.6366) (-31.4955, 30.6807) (-31.4985, 30.7248) (-31.5016, 30.7689) (-31.5049, 30.8131) (-31.5084, 30.8573) (-31.5121, 30.9015) (-31.5159, 30.9458) (-31.52, 30.99) (-31.5242, 31.0343) (-31.5286, 31.0787) (-31.5331, 31.123) (-31.5379, 31.1674) (-31.5428, 31.2118) (-31.5479, 31.2562) (-31.5531, 31.3006) (-31.5585, 31.3451) (-31.5641, 31.3895) (-31.5699, 31.434) (-31.5758, 31.4785) (-31.5819, 31.523) (-31.5881, 31.5676) (-31.5946, 31.6122) (-31.6011, 31.6567) (-31.6079, 31.7013) (-31.6148, 31.7459) (-31.6218, 31.7906) (-31.629, 31.8352) (-31.6349, 31.8709) (-31.6394, 31.8977) (-31.6424, 31.9156) (-31.644, 31.9245) knots 0.354152 0.354152 0.354152 0.354152 0.354152 0.354152 0.357143 0.371429 0.385714 0.4 0.414286 0.428571 0.442857 0.457143 0.471429 0.485714 0.5 0.514286 0.528571 0.542857 0.557143 0.571429 0.585714 0.6 0.614286 0.628571 0.642857 0.657143 0.671429 0.685714 0.7 0.714286 0.728571 0.742857 0.757143 0.771429 0.785714 0.8 0.814286 0.828571 0.842857 0.857143 0.871429 0.885714 0.9 0.914286 0.928571 0.942857 0.957143 0.971429 0.985714 1 1 1 1 1 1
  arc A93 (-31.644, 31.9245) -> (-32.3342, 32.0973) centre (-40, 0) ccw
  spline S186 degree 5 poles (-32.3342, 32.0973) (-32.3398, 32.0901) (-32.3509, 32.0758) (-32.3675, 32.0543) (-32.3895, 32.0255) (-32.4169, 31.9895) (-32.4441, 31.9535) (-32.4712, 31.9174) (-32.4982, 31.8812) (-32.525, 31.845) (-32.5516, 31.8087) (-32.5781, 31.7724) (-32.6044, 31.7359) (-32.6306, 31.6995) (-32.6567, 31.6629) (-32.6825, 31.6263) (-32.7083, 31.5897) (-32.7338, 31.553) (-32.7592, 31.5162) (-32.7845, 31.4793) (-32.8095, 31.4424) (-32.8345, 31.4055) (-32.8592, 31.3684) (-32.8838, 31.3314) (-32.9082, 31.2942) (-32.9324, 31.257) (-32.9565, 31.2197) (-32.9804, 31.1824) (-33.0041, 31.145) (-33.0277, 31.1075) (-33.051, 31.07) (-33.0742, 31.0324) (-33.0972, 30.9947) (-33.1201, 30.957) (-33.1427, 30.9192) (-33.1651, 30.8814) (-33.1874, 30.8434) (-33.2095, 30.8055) (-33.2313, 30.7674) (-33.253, 30.7293) (-33.2745, 30.6911) (-33.2957, 30.6529) (-33.3168, 30.6146) (-33.3376, 30.5762) (-33.3583, 30.5378) (-33.3787, 30.4992) (-33.3957, 30.4668) (-33.4085, 30.442) (-33.4173, 30.4249) (-33.4221, 30.4155) (-33.4229, 30.4139) knots -1 -1 -1 -1 -1 -1 -0.985714 -0.971429 -0.957143 -0.942857 -0.928571 -0.914286 -0.9 -0.885714 -0.871429 -0.857143 -0.842857 -0.828571 -0.814286 -0.8 -0.785714 -0.771429 -0.757143 -0.742857 -0.728571 -0.714286 -0.7 -0.685714 -0.671429 -0.657143 -0.642857 -0.628571 -0.614286 -0.6 -0.585714 -0.571429 -0.557143 -0.542857 -0.528571 -0.514286 -0.5 -0.485714 -0.471429 -0.457143 -0.442857 -0.428571 -0.414286 -0.4 -0.385714 -0.371429 -0.357143 -0.354152 -0.354152 -0.354152 -0.354152 -0.354152 -0.354152
  spline S187 degree 3 poles (-33.9662, 30.1514) (-33.9023, 30.1386) (-33.8366, 30.1384) (-33.7088, 30.1633) (-33.6479, 30.188) (-33.5575, 30.2475) (-33.5247, 30.2757) (-33.4671, 30.3399) (-33.4426, 30.3755) (-33.4229, 30.4139) knots 0 0 0 0 0.019532 0.019532 0.039064 0.039064 0.051994 0.051994 0.064924 0.064924 0.064924 0.064924
  arc A94 (-33.9662, 30.1514) -> (-34.0493, 30.1679) centre (-40, 0) ccw
  spline S188 degree 3 poles (-34.4509, 30.6181) (-34.4456, 30.5532) (-34.4277, 30.49) (-34.3688, 30.3739) (-34.3282, 30.3222) (-34.2462, 30.2515) (-34.2101, 30.2277) (-34.1326, 30.19) (-34.0915, 30.1762) (-34.0493, 30.1679) knots 0 0 0 0 0.019532 0.019532 0.039064 0.039064 0.051994 0.051994 0.064924 0.064924 0.064924 0.064924